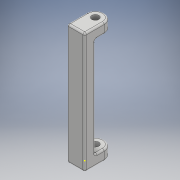
# Autodesk Inventor part: support
Saved by Autodesk Inventor 2018 (Build 220112000, 112)
## iProperties
Created: 2018-04-27
Part Number: support
Material: Generic
Document SubType Name: Modeling
Designer: Matyi
Density: 1 g/cm^3
Appearance: Default
Author: Matyi
Autodesk Inventor part; units mm, degrees
ref_plane "YZ Plane" through (0, 0, 0) normal (1, 0, 0) x (0, 1, 0)
ref_plane "XZ Plane" through (0, 0, 0) normal (0, 1, 0) x (-1, 0, 0)
ref_plane "XY Plane" through (0, 0, 0) normal (0, 0, 1) x (1, 0, 0)
sketch "Sketch1" plane through (0, 0, 0) normal (0, 1, 0) x (-1, 0, 0)
  line L0 (0, 0) -> (5, 0)
  line L1 (5, 0) -> (5, -34)
  line L2 (5, -34) -> (0, -34)
  line L3 (0, -34) -> (0, 0)
  dimension "d0" = 5
  dimension "d1" = 34
  constraints: 8 end point, 2 parallel, 1 horizontal, 1 perpendicular
  measures "d0" distance of L1.end L2.end
  measures "d1" distance of L0.end L1.end
extrude "Extrusion1" add sketch "Sketch1" along normal blind 3
sketch "Sketch2" plane through (0, 3, 0) normal (0, 1, 0) x (1, 0, 0)
  line L0 (-5, 0) -> (0, 0) projected
  line L1 (-5, 34) -> (-5, 0) projected
  line L2 (0, 0) -> (-5, 0)
  line L3 (-5, 0) -> (-5, 3)
  line L4 (-5, 3) -> (0, 3)
  line L5 (0, 3) -> (0, 0)
  line L6 (0, 34) -> (-5, 34) projected
  line L7 (-5, 34) -> (0, 34)
  line L8 (0, 34) -> (0, 31)
  line L9 (0, 31) -> (-5, 31)
  line L10 (-5, 31) -> (-5, 34)
  dimension "d4" = 3
  dimension "d5" = 5
  dimension "d6" = 3
  constraints: 16 end point, 4 parallel, 2 horizontal, 2 perpendicular, 1 point on line
  measures "d4" distance of L2.end L3.end
  measures "d5" distance of L8.end L9.end
  measures "d6" distance of L7.end L8.end
extrude "Extrusion2" add sketch "Sketch2" along normal blind 5
fillet "Fillet1" radius 2.5 4 edges at (0, 8, -1.5) (-5, 8, -1.5) (-5, 8, -32.5) (0, 8, -32.5)
sketch "Sketch3" plane through (-5, 3, -31) normal (0, 0, 1) x (1, 0, 0)
  point P0 (5, -3)
sketch "Sketch4" plane through (-5, 0, 0) normal (0, 0, 1) x (1, 0, 0)
  circle A0 centre (2.5, 5.5) radius 1
  arc A1 (5, 5.5) -> (0, 5.5) centre (2.5, 5.5) ccw projected
  line L0 (5, 0) -> (5, 5.5) projected
  dimension "d10" = 2
  dimension "d11" = 0
  dimension "d12" = 2.5
  constraints: 1 centre point
  measures "d10" diameter of A0
  measures "d11" distance of A1.centre A0.centre
  measures "d12" distance from line of L0 A0.centre
sketch "Sketch5" plane through (0, 0, -34) normal (0, 0, -1) x (-1, 0, 0)
  circle A0 centre (2.5, 5.5) radius 1
  arc A1 (5, 5.5) -> (0, 5.5) centre (2.5, 5.5) ccw projected
  line L0 (5, 0) -> (5, 5.5) projected
  point P0 (0, 0)
  dimension "d13" = 2
  dimension "d14" = 0
  dimension "d15" = 2.5
  constraints: 1 centre point
  measures "d13" diameter of A0
  measures "d14" distance of A1.centre A0.centre
  measures "d15" distance from line of A0.centre L0
extrude "Extrusion3" cut sketch "Sketch5" against normal blind 3
extrude "Extrusion4" cut sketch "Sketch4" against normal blind 3
fillet "Fillet2" radius 0.5 20 edges at (-4.2679, 7.2679, -34) (-5, 2.7503, -34) (0, 2.7503, -34) (-4.2679, 7.2679, -31) (-5, 4.2503, -31) (0, 4.2503, -31) (0, 3, -17) (0, 0, -17) (-2.5, 0, -34) (-0.7321, 7.2679, -3) (-5, 4.2503, -3) (0, 4.2503, -3) (-0.7321, 7.2679, 0) (-5, 2.7503, 0) (0, 2.7503, 0) (-2.5, 3, -3) (-5, 3, -17) (-5, 0, -17) (-2.5, 0, 0) (-2.5, 3, -31)
body "Solid1"
